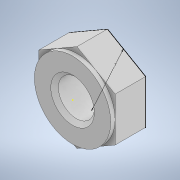
# Autodesk Inventor part: nakretka
Saved by Autodesk Inventor 2020 (Build 240168000, 168)
## iProperties
Created: 2020-03-28
Part Number: nakretka
Material: Ogólny
Document SubType Name: Modeling
Designer: niedz
Density: 1 g/cm^3
Appearance: Domyślna
Author: niedz
Autodesk Inventor part; units mm, degrees
ref_plane "YZ Plane" through (0, 0, 0) normal (1, 0, 0) x (0, 1, 0)
ref_plane "XZ Plane" through (0, 0, 0) normal (0, 1, 0) x (-1, 0, 0)
ref_plane "XY Plane" through (0, 0, 0) normal (0, 0, 1) x (1, 0, 0)
sketch "Szkic1" plane through (0, 0, 0) normal (0, 0, 1) x (1, 0, 0)
  circle A0 centre (0, 0) radius 3.5
  circle A1 centre (0, 0) radius 1.65
  dimension "d0" = 7
  dimension "d1" = 3.3
  constraints: 2 centre point, 2 coincident
  measures "d0" diameter of A0
  measures "d1" diameter of A1
extrude "Wyciągnięcie proste1" add sketch "Szkic1" along normal blind 0.4
chamfer "Faza1" distance 0.35 angle 45 1 edges at (-1.65, 0, 0.4)
sketch "Szkic2" plane through (0, 0, 0.4) normal (0, 0, 1) x (1, 0, 0)
  point P0 (0, 0)
sketch "Szkic3" plane through (0, 0, 0) normal (0, 0, -1) x (-1, 0, 0)
  circle A0 centre (0, 0) radius 1.65
  circle A1 centre (0, 0) radius 3.5
  circle A2 centre (0, 0) radius 3.5 projected
  line L0 (1.75, 3.0311) -> (3.5, 2.0207)
  line L1 (1.75, 3.0311) -> (0, 4.0415)
  line L2 (-1.75, 3.0311) -> (0, 4.0415)
  line L3 (-1.75, 3.0311) -> (-3.5, 2.0207)
  line L4 (-3.5, 0) -> (-3.5, 2.0207)
  line L5 (-3.5, 0) -> (-3.5, -2.0207)
  line L6 (-1.75, -3.0311) -> (-3.5, -2.0207)
  line L7 (-1.75, -3.0311) -> (0, -4.0415)
  line L8 (0, -4.0415) -> (1.75, -3.0311)
  line L9 (1.75, -3.0311) -> (3.5, -2.0207)
  line L10 (3.5, 0) -> (3.5, -2.0207)
  line L11 (3.5, 0) -> (3.5, 2.0207)
  constraints: 24 end point, 4 vertical, 2 centre point, 2 coincident, 2 point on line, 1 horizontal alignment, 1 tangent, 3 other
extrude "Wyciągnięcie proste2" add sketch "Szkic3" along normal blind 2.8 contours A0 | A1 | L10 L9 A1 | A1 L0 L11 | A1 L2 L1 | L8 L7 A1 | A1 L4 L3 | L6 L5 A1
sketch "Szkic4" plane through (0, 0, 0) normal (0, 0, 1) x (1, 0, 0)
  circle A0 centre (0, 0) radius 1.65
  constraints: 1 centre point, 1 coincident
extrude "Wyciągnięcie proste3" cut sketch "Szkic4" against normal blind 2.8
chamfer "Faza2" distance 0.35 angle 45 1 edges at (-1.65, 0, -2.8)
sketch "Szkic5" plane through (0, 0, -2.8) normal (0, 0, -1) x (-1, 0, 0)
  circle A0 centre (0, 0) radius 3.5
  dimension "d18" = 7
  constraints: 1 centre point, 1 coincident
  measures "d18" diameter of A0
sketch "Szkic6" plane through (0, 0, -2.8) normal (0, 0, -1) x (-1, 0, 0)
  line L0 (-3.5, 2.0207) -> (-3.5, -2.0207) projected
  line L1 (-3.5, -2.0207) -> (-3.5, 0)
  line L2 (-3.5, 2.0207) -> (-3.5, 0) projected
  line L3 (-3.5, 0) -> (-3.5, 2.0207)
  line L4 (-3.5, 2.0207) -> (-1.75, 3.0311)
  line L5 (0, 4.0415) -> (-3.5, 2.0207) projected
  line L6 (-1.75, 3.0311) -> (0, 4.0415)
  line L7 (0, 4.0415) -> (1.75, 3.0311)
  line L8 (3.5, 2.0207) -> (0, 4.0415) projected
  line L9 (1.75, 3.0311) -> (3.5, 2.0207)
  line L10 (3.5, 2.0207) -> (3.5, 0)
  line L11 (3.5, -2.0207) -> (3.5, 0) projected
  line L12 (3.5, 0) -> (3.5, -2.0207)
  arc A0 (-1.75, -3.0311) -> (1.75, -3.0311) centre (0, 0) ccw projected
  line L13 (3.5, -2.0207) -> (1.75, -3.0311)
  line L14 (-3.5, -2.0207) -> (0, -4.0415) projected
  line L15 (1.75, -3.0311) -> (0, -4.0415)
  line L16 (0, -4.0415) -> (-1.75, -3.0311)
  arc A1 (-3.5, 0) -> (-1.75, -3.0311) centre (0, 0) ccw projected
  line L17 (-1.75, -3.0311) -> (-3.5, -2.0207)
  constraints: 24 end point, 5 collinear, 4 midpoint, 2 parallel, 2 tangent, 1 vertical
sketch "Szkic7" plane through (0, 0, -2.8) normal (0, 0, -1) x (-1, 0, 0)
  point P0 (0, 0)
